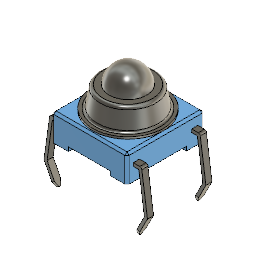
3347 metal ball button (Autodesk Fusion 360 design; units mm, degrees)
Autodesk Fusion 360 part; units mm, degrees
sketch "Sketch1" plane through (0, 0, 0) normal (0, 0, 1) x (1, 0, 0)
  line L0 (3.6, 3.7) -> (-3.6, 3.7)
  line L1 (-3.6, 3.7) -> (-3.6, -3.7)
  line L2 (-3.6, -3.7) -> (3.6, -3.7)
  line L3 (3.6, -3.7) -> (3.6, 3.7)
  line L4 (3.6, 3.7) -> (-3.6, -3.7) construction
  line L5 (-3.6, 3.7) -> (3.6, -3.7) construction
  circle A0 centre (0, 0) radius 2.6
  circle A1 centre (0, 0) radius 1.9
  circle A2 centre (0, 0) radius 3.4
  dimension "d1" = 7.2
  dimension "d2" = 7.4
  dimension "d3" = 5.2
  dimension "d4" = 3.8
  dimension "d41" = 6.8
  measures "d3" diameter of A0
  measures "d4" diameter of A1
  measures "d41" diameter of A2
extrude "Extrude1" add sketch "Sketch1" against normal blind 2.6 contours L0 L1 L2 L3 | A0 | A1 | A2 makes body 1
extrude "Extrude2" add sketch "Sketch1" along normal blind 2.15 separate body contours A0 | A1 makes body 2
sphere "SpherePrimitive1" add diameter 3.6 placed x (-1, 0, 0) y (0, -1, 0) z (0, 0, 1) at (0, 0, 2.15) bodies 2 1
fillet "Fillet1" [suppressed]
sketch "Sketch3" plane through (0, 0, 0) normal (0, 1, 0) x (1, 0, 0)
  line L0 (-3.6, 0) -> (-3.6, 2.6)
  line L1 (-3.6, 1) -> (-4.4, 1)
  line L2 (-4.4, 1) -> (-4.9625, 5.0024)
  line L3 (-4.9625, 5.0024) -> (-3.9956, 6.9)
  line L4 (-3.6, 1.3) -> (-4.1392, 1.3)
  line L5 (-4.1392, 1.3) -> (-4.6523, 4.9505)
  line L6 (-4.6523, 4.9505) -> (-3.7283, 6.7638)
  line L7 (-3.7283, 6.7638) -> (-3.9956, 6.9)
  dimension "d11" = 98
  dimension "d12" = 145
  dimension "d13" = 0.3
  dimension "d14" = 0.3
  dimension "d15" = 0.3
  dimension "d16" = 0.8
  dimension "d17" = 5.9
  dimension "d18" = 1
  measures "d11" angle of L1 L2
  measures "d12" angle of L2 L3
  measures "d13" distance of L3 L6
  measures "d14" distance of L2 L5
  measures "d15" distance of L1 L4
  measures "d17" distance of L1
extrude "Extrude3" add sketch "Sketch3" along normal blind 0.6 from surface at 2.5 separate body makes body 3
fillet "Fillet2" radius 0.2 1 edges at (-4.4, 2.8, -1) on bodies 3
fillet "Fillet3" radius 0.1 1 edges at (-4.1392, 2.8, -1.3) on bodies 3
chamfer "Chamfer1" distance 0.5 angle 22 1 edges at (-3.862, 3.1, -6.8319) measured on face at (-4.5127, 3.1, -2.5202) on bodies 3
chamfer "Chamfer2" distance 0.2 angle 70 1 edges at (-3.862, 2.5, -6.8319) measured on face at (-3.8174, 2.6327, -6.8092) on bodies 3
mirror "Mirror1" about plane through (0, 0, 0) normal (0, 1, 0) of bodies 3 makes body 4
mirror "Mirror2" about plane through (0, 0, 0) normal (1, 0, 0) of bodies 3 4 makes body 5 at (4.6036, 2.7, -2.4489) makes body 6 at (4.6036, -2.7, -2.4489)
sketch "Sketch4" plane through (0, -3.7, 0) normal (0, -1, 0) x (1, 0, 0)
  line L0 (3.6, 0) -> (-3.6, 0)
  line L1 (-3.6, 0) -> (-3.6, -2.6)
  line L2 (-3.6, -2.6) -> (3.6, -2.6)
  line L3 (3.6, -2.6) -> (3.6, 0)
  line L4 (-2, -2.2) -> (2, -2.2)
  line L5 (2, -2.2) -> (2, -2.6)
  line L6 (2, -2.6) -> (-2, -2.6)
  line L7 (-2, -2.6) -> (-2, -2.2)
  dimension "d30" = 4
  dimension "d31" = 0.4
extrude "Extrude4" cut sketch "Sketch4" against normal up to surface (7.4 mm away) contours L2 L4 L5 L6 L7 bodies 1
sketch "Sketch5" plane through (-3.6, 0, 0) normal (-1, 0, 0) x (0, -1, 0)
  line L0 (3.7, 0) -> (-3.7, 0)
  line L1 (-3.7, 0) -> (-3.7, -2.6)
  line L2 (-3.7, -2.6) -> (3.7, -2.6)
  line L3 (3.7, -2.6) -> (3.7, 0)
  line L4 (-2, -2.2) -> (2, -2.2)
  line L5 (2, -2.2) -> (2, -2.6)
  line L6 (2, -2.6) -> (-2, -2.6)
  line L7 (-2, -2.6) -> (-2, -2.2)
  dimension "d34" = 0.4
  dimension "d35" = 4
extrude "Extrude5" cut sketch "Sketch5" against normal up to surface (7.2 mm away) contours L2 L4 L5 L6 L7 bodies 1
draft "Draft1" angle 10 neutral plane through (0, 0, 2.15) pull (0, 0, 1) 1 faces at (2.5871, -0.2589, 1.4333) on bodies 2
fillet "Fillet4" radius 0.3 1 edges at (-2.4241, -0.9402, 2.15) on bodies 2
extrude "Extrude6" add sketch "Sketch1" along normal blind 0.2 contours A2 bodies 2
fillet "Fillet5" radius 0.2 1 edges at (-2.7446, -1.0645, 0.2) on bodies 2
chamfer "Chamfer3" distance 0.2 angle 45 8 edges at (0, 3.7, 0) (0, -3.7, 0) (-3.6, 0, 0) (-3.6, -3.7, -1.3) (-3.6, 3.7, -1.3) (3.6, 3.7, -1.3) (3.6, -3.7, -1.3) (3.6, 0, 0) measured on face at (-1.2, 1.2333, 0) measured on face at (-1.2, 1.2333, 0) measured on face at (-1.2, 1.2333, 0) measured on face at (-0.6667, -3.7, -0.7333) measured on face at (-3.6, 0.6667, -0.7333) measured on face at (0.6667, 3.7, -0.7333) measured on face at (3.6, -0.6667, -0.7333) measured on face at (-1.2, 1.2333, 0) on bodies 1
equation "d9 = ( 1.8 * 2 ) * 1 mm"
